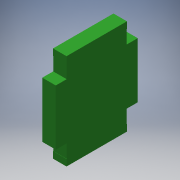
# Autodesk Inventor part: arpm4_14
Saved by Autodesk Inventor 2016 (Build 200138000, 138)
## iProperties
Created: 2017-09-25
Part Number: arpm4_14
Material: Generic
Document SubType Name: Modeling
Designer: student
Density: 1 g/cm^3
Appearance: Default
Author: student
Autodesk Inventor part; units mm, degrees
ref_plane "YZ Plane" through (0, 0, 0) normal (1, 0, 0) x (0, 1, 0)
ref_plane "XZ Plane" through (0, 0, 0) normal (0, 1, 0) x (-1, 0, 0)
ref_plane "XY Plane" through (0, 0, 0) normal (0, 0, 1) x (1, 0, 0)
sketch "Sketch1" plane through (0, 0, 0) normal (1, 0, 0) x (0, 1, 0)
  line L0 (-5.5858, -44.087) -> (-8.4893, -44.087)
  line L1 (-8.4893, -44.087) -> (-8.4893, -44.1249)
  line L2 (-8.4893, -44.1249) -> (-9.9094, -44.1249)
  line L3 (-9.9094, -44.1249) -> (-9.9094, -31.0439)
  line L4 (6.4385, -44.087) -> (9.342, -44.087)
  line L5 (9.342, -44.087) -> (9.342, -44.1249)
  line L6 (9.2388, -31.0818) -> (9.2388, -31.0822)
  line L7 (9.342, -44.1249) -> (10.7622, -44.1249)
  line L8 (10.7622, -44.1249) -> (10.7622, -31.0439)
  line L9 (-5.5858, -31.0439) -> (-5.5858, -28.7148)
  line L10 (-5.5858, -44.087) -> (-5.5858, -46.454)
  line L11 (-5.5858, -28.7148) -> (6.4385, -28.7148)
  line L12 (6.4385, -44.087) -> (6.4385, -46.454)
  line L13 (6.4385, -46.454) -> (-5.5858, -46.454)
  line L14 (-5.5858, -31.0818) -> (-5.5858, -31.0439)
  line L15 (-9.0353, -37.5844) -> (-13.1011, -37.5844) construction
  line L16 (-5.5858, -31.0818) -> (-8.4893, -31.0818)
  line L17 (-8.4893, -31.0818) -> (-8.4893, -31.0439)
  line L18 (-8.4893, -31.0439) -> (-9.9094, -31.0439)
  line L19 (6.4385, -31.0818) -> (9.342, -31.0818)
  line L20 (9.342, -31.0818) -> (9.342, -31.0439)
  line L21 (9.342, -31.0439) -> (10.7622, -31.0439)
  line L22 (6.4385, -31.0818) -> (6.4385, -28.7148)
  point P0 (0, 0)
  dimension "d17" = 13.081
  constraints: 47 end point, 7 symmetric about line, 4 horizontal, 3 vertical, 2 perpendicular
  measures "d17" distance of L2.end L3.end
extrude "Extrusion1" add sketch "Sketch1" along normal blind 2.921
body "Solid1"
